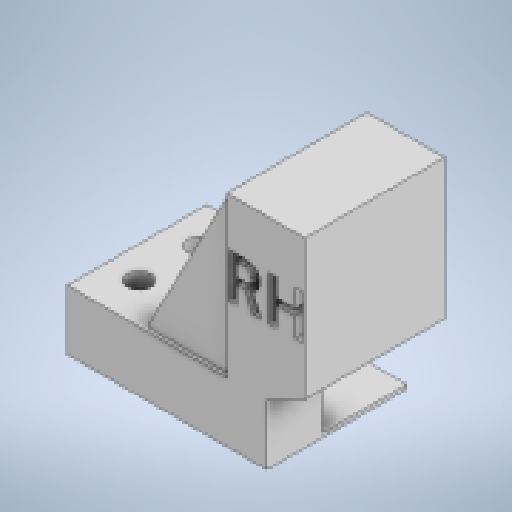
# Autodesk Inventor part: gripper
Saved by Autodesk Inventor 2024 (Build 280153000, 153)
## iProperties
Created: 2023-09-08
Part Number: gripper
Material: Generic
Document SubType Name: Modeling
Designer: 박동준
Density: 1 g/cm^3
Appearance: Default
Author: 박동준
Autodesk Inventor part; units mm, degrees
ref_plane "YZ Plane" through (0, 0, 0) normal (1, 0, 0) x (0, 1, 0)
ref_plane "XZ Plane" through (0, 0, 0) normal (0, 1, 0) x (-1, 0, 0)
sketch "Sketch1" plane through (0, 0, 0) normal (0, 0, 1) x (1, 0, 0)
  line L0 (-10, 40) -> (-10, 0)
  line L1 (-10, 0) -> (0, 0)
  line L2 (0, 0) -> (9.5, 5)
  line L3 (9.5, 5) -> (9.5, 40)
  line L4 (9.5, 40) -> (-10, 40)
  dimension "d0" = 40
  dimension "d2" = 10
  dimension "d55" = 9.5
  dimension "d57" = 35
  constraints: 10 end point, 2 perpendicular, 1 parallel, 1 vertical
  measures "d0" distance of L0.start L0.end
  measures "d2" distance of L0.end L1.end
  measures "d55" distance from line of L3 L1.end
  measures "d57" distance of L2.end L3.end
extrude "Extrusion1" add sketch "Sketch1" along normal mid plane 35
ref_plane "Work Plane1" through (0, 0, 15) normal (0, 0, 1) x (1, 0, 0)
sketch "Sketch2" plane through (0, 0, 15) normal (0, 0, 1) x (1, 0, 0)
  line L0 (-10, 40) -> (-10, 0) projected
  line L1 (-10, 0) -> (0, 0) projected
  line L2 (-10, 0) -> (-31, 0)
  line L3 (-10, 0) -> (11, 0) construction
  line L4 (0, 0) -> (9.5, 5) projected
  line L5 (9.5, 5) -> (9.5, 40) projected
  line L6 (9.5, 40) -> (-10, 40) projected
  line L7 (-31, 0) -> (-10, 40)
  line L8 (-10, 0) -> (-10, 40)
  dimension "d9" = 21
  dimension "d10" = 180
  dimension "d88" = 40
  constraints: 8 end point, 2 collinear, 2 horizontal, 1 point on line
  measures "d9" distance of L0.end L2.end
  measures "d10" angle of L2 L3
  measures "d88" distance from line of L1 L7.end
extrude "Extrusion2" add sketch "Sketch2" along normal mid plane 3 contours L0 L2 L7
mirror "Mirror1" about plane through (0, 0, 0) normal (0, 0, 1) of "Extrusion2"
sketch "Sketch3" plane through (-10, 0, 17.5) normal (0, -1, 0) x (1, 0, 0)
  line L0 (-40, 2) -> (-15.2727, 11)
  line L1 (-15.2727, 11) -> (10, 11)
  line L2 (10, 11) -> (10, -46)
  line L3 (-40, 2) -> (-40, -37)
  line L4 (-40, -37) -> (-15.2727, -46)
  line L5 (-15.2727, -46) -> (10, -46)
  line L6 (10, -35) -> (10, 0) projected
  line L7 (10, -35) -> (10, 0) projected
  line L8 (0, 0) -> (0, -1) projected
  line L9 (10, -35) -> (0, -35) projected
  line L10 (0, 0) -> (10, 0) projected
  line L11 (-21, -1) -> (0, -1) projected
  line L12 (-21, -4) -> (-21, -1) projected
  line L13 (0, -4) -> (-21, -4) projected
  line L14 (0, -4) -> (0, -31) projected
  line L15 (0, -31) -> (-21, -31) projected
  line L16 (-21, -31) -> (-21, -34) projected
  line L17 (-21, -34) -> (0, -34) projected
  line L18 (0, -34) -> (0, -35) projected
  point P0 (10, -17.5)
  point P1 (-2.6364, 11)
  point P2 (10, -17.5)
  point P3 (10, -17.5)
  point P4 (10, -17.5)
  point P5 (-2.6364, -46)
  point P6 (-40, -17.5)
  point P7 (10, -17.5)
  point P8 (10, -35)
  point P9 (10, 0)
  dimension "d17" = 57
  dimension "d18" = 39
  dimension "d19" = 9
  dimension "d20" = 9
  dimension "d21" = 50
  dimension "d76" = 110
  constraints: 12 end point, 7 midpoint, 3 coincident, 1 horizontal alignment, 1 perpendicular, 1 vertical alignment
  measures "d17" distance of L1.end L2.end
  measures "d18" distance of L0.start L3.end
  measures "d19" distance from line of L5 L3.end
  measures "d20" vertical distance of point (-2.636, 11) L0.start
  measures "d21" distance between parallel lines of L2 L3
  measures "d76" angle of L3 L4
extrude "Extrusion3" add sketch "Sketch3" along normal blind 15
sketch "Sketch4" plane through (-10, 0, 17.5) normal (0, 1, 0) x (1, 0, 0)
  line L0 (10, 17.5) -> (-48, 17.5) construction
  line L1 (-32, 10) -> (-12, 10) construction
  line L2 (-32, 25) -> (-32, 10) construction
  line L3 (10, 35) -> (0, 35) projected
  line L4 (10, 46) -> (10, 35) projected
  line L5 (-15.2727, 46) -> (10, 46) projected
  line L6 (-40, 37) -> (-15.2727, 46) projected
  line L7 (-40, -2) -> (-40, 37) projected
  line L8 (-15.2727, -11) -> (-40, -2) projected
  line L9 (10, -11) -> (-15.2727, -11) projected
  line L10 (10, 0) -> (10, -11) projected
  line L11 (0, 0) -> (10, 0) projected
  line L12 (0, 0) -> (0, 1) projected
  line L13 (-21, 1) -> (0, 1) projected
  line L14 (-21, 4) -> (-21, 1) projected
  line L15 (0, 4) -> (-21, 4) projected
  line L16 (0, 4) -> (0, 31) projected
  line L17 (0, 31) -> (-21, 31) projected
  line L18 (-21, 31) -> (-21, 34) projected
  line L19 (-21, 34) -> (0, 34) projected
  line L20 (0, 34) -> (0, 35) projected
  point P0 (-32, 17.5)
  point P1 (-19, 17.5)
  dimension "d26" = 20
  dimension "d27" = 15
  dimension "d58" = 13
  dimension "d59" = 8
  constraints: 6 end point, 2 horizontal, 2 midpoint, 2 perpendicular, 1 horizontal alignment
  measures "d26" distance of L1.end L1.start
  measures "d27" distance of L2.start L1.start
  measures "d58" distance from line of L2 point (-19, 17.5)
  measures "d59" distance from line of point (-32, 17.5) L7
hole "Hole1" at (-42, 0, 7.5) at (-22, 0, 7.5) at (-42, 0, -7.5) direction (0, -1, 0) diameter 3.1 end through all
sketch "Sketch5" plane through (0, 0, -17.5) normal (1, 0, 0) x (0, 0, -1)
  line L0 (11, 0) -> (0, 0) projected
  line L1 (-35, 0) -> (-46, 0) projected
  line L2 (-46, 0) -> (-46, -15) projected
  line L3 (11, -15) -> (-46, -15) projected
  line L4 (11, 0) -> (11, -15) projected
  line L5 (-46, 0) -> (-46, -15) projected
  line L6 (-21, -4) -> (9, -4)
  line L7 (9, -4) -> (9, -14)
  line L8 (9, -14) -> (-21, -14)
  line L9 (-21, -14) -> (-21, -4)
  line L10 (0, 0) -> (-35, 0) projected
  point P0 (-17.5, 0)
  point P1 (-17.5, 0)
  point P2 (-46, -7.5)
  point P3 (-46, -7.5)
  point P4 (11, -12.5)
  point P5 (11, -2.5)
  dimension "d46" = 30
  dimension "d47" = 10
  dimension "d48" = 2
  dimension "d49" = 4
  constraints: 8 end point, 2 midpoint, 2 parallel
  measures "d46" distance of L7.end L8.end
  measures "d47" distance of L6.end L7.end
  measures "d48" distance between parallel lines of L4 L7
  measures "d49" distance between parallel lines of L6 L0
extrude "Extrusion4" cut sketch "Sketch5" against normal blind 30 contours L6 L7 L8 L9
sketch "Sketch6" plane through (-10, 0, 17.5) normal (0, 1, 0) x (1, 0, 0)
  circle A0 centre (-32, 25) radius 1.55 projected
  circle A1 centre (-12, 10) radius 1.55 projected
  circle A2 centre (-32, 10) radius 1.55 projected
  line L0 (10, 35) -> (0, 35) projected
  line L1 (10, 46) -> (10, 35) projected
  line L2 (-15.2727, 46) -> (10, 46) projected
  line L3 (-40, 37) -> (-15.2727, 46) projected
  line L4 (-40, -2) -> (-40, 37) projected
  line L5 (-15.2727, -11) -> (-40, -2) projected
  line L6 (10, -11) -> (-15.2727, -11) projected
  line L7 (10, 0) -> (10, -11) projected
  line L8 (0, 0) -> (10, 0) projected
  line L9 (0, 0) -> (0, 1) projected
  circle A3 centre (-12, 25) radius 2.9
  line L10 (-21, 1) -> (0, 1) projected
  line L11 (-21, 4) -> (-21, 1) projected
  line L12 (0, 4) -> (-21, 4) projected
  line L13 (0, 4) -> (0, 31) projected
  line L14 (0, 31) -> (-21, 31) projected
  line L15 (-21, 31) -> (-21, 34) projected
  line L16 (-21, 34) -> (0, 34) projected
  line L17 (0, 34) -> (0, 35) projected
  point P0 (10, 17.5)
  dimension "d41" = 5.8
  dimension "d42" = 20
  dimension "d43" = 15
  constraints: 1 centre point
  measures "d41" diameter of A3
  measures "d42" distance of A3.centre A0.centre
  measures "d43" distance of A3.centre A1.centre
extrude "Extrusion5" cut sketch "Sketch6" against normal blind 3 contours A3
sketch "Sketch7" plane through (-10, -15, 17.5) normal (0, -1, 0) x (1, 0, 0)
  circle A0 centre (-12, -25) radius 1.55
  circle A1 centre (-32, -25) radius 1.55 projected
  circle A2 centre (-12, -10) radius 1.55 projected
  circle A3 centre (-32, -10) radius 1.55 projected
  line L0 (10, -46) -> (10, 11) projected
  line L1 (10, 11) -> (-15.2727, 11) projected
  line L2 (-15.2727, 11) -> (-40, 2) projected
  line L3 (-40, 2) -> (-40, -37) projected
  line L4 (-40, -37) -> (-15.2727, -46) projected
  line L5 (-15.2727, -46) -> (10, -46) projected
  point P0 (10, -17.5)
  dimension "d50" = 15
  dimension "d51" = 20
  dimension "d52" = 3.1
  constraints: 1 centre point
  measures "d50" distance of A0.centre A2.centre
  measures "d51" distance of A1.centre A0.centre
  measures "d52" diameter of A0
extrude "Extrusion6" cut sketch "Sketch7" against normal up to surface (1 mm away) contours A0
sketch "Sketch8" plane through (0, 0, 17.5) normal (0, 0, 1) x (1, 0, 0)
  line L0 (-10, 0) -> (0, 0) projected
  line L1 (0, 0) -> (9.5, 5) projected
  line L2 (9.5, 5) -> (9.5, 40) projected
  line L3 (9.5, 40) -> (-10, 40) projected
  line L4 (-10, 40) -> (-10, 0) projected
  line L5 (-10.7901, 28) -> (5, 28) construction
  line L6 (5, 28) -> (5, 11.9362) construction
  line L7 (5, 11.9362) -> (-10.7901, 11.9362) construction
  line L8 (-10.7901, 11.9362) -> (-10.7901, 28) construction
  line L9 (-5.3559, 21.4049) -> (-7.6037, 21.4049)
  line L10 (-7.6037, 21.4049) -> (-7.6037, 17)
  line L11 (-7.6037, 17) -> (-9.555, 17)
  line L12 (-9.555, 17) -> (-9.555, 28)
  line L13 (-9.555, 28) -> (-5.3889, 28)
  spline S0 degree 2 poles (-5.3889, 28) (-4.5326, 28) (-3.207, 27.5389) (-2.3095, 26.7485) (-1.832, 25.637) (-1.832, 24.9783) knots 0 0 0 1 2 3 4 4 4
  line L14 (-1.832, 24.9783) -> (-1.832, 24.4102)
  spline S1 degree 2 poles (-1.832, 24.4102) (-1.832, 23.5457) (-2.6883, 22.1542) (-3.5445, 21.7754) knots 0 0 0 1 2 2 2
  spline S2 degree 2 poles (-3.5445, 21.7754) (-2.9929, 20.5651) (-1.939, 18.2021) (-1.3956, 17) knots 0 0 0 1 2 2 2
  line L15 (-1.3956, 17) -> (-3.5116, 17)
  line L16 (-3.5116, 17) -> (-5.3559, 21.4049)
  line L17 (-7.6037, 26.3698) -> (-7.6037, 23.0434)
  line L18 (-7.6037, 23.0434) -> (-5.8005, 23.0434)
  spline S3 degree 2 poles (-5.8005, 23.0434) (-4.6725, 23.0434) (-3.7751, 23.8338) (-3.7751, 24.4596) knots 0 0 0 1 2 2 2
  line L19 (-3.7751, 24.4596) -> (-3.7751, 24.9207)
  spline S4 degree 2 poles (-3.7751, 24.9207) (-3.7751, 25.5546) (-4.6231, 26.3698) (-5.6359, 26.3698) knots 0 0 0 1 2 2 2
  line L20 (-5.6359, 26.3698) -> (-7.6037, 26.3698)
  line L21 (7.0273, 21.9237) -> (2.4659, 21.9237)
  line L22 (2.4659, 21.9237) -> (2.4659, 17)
  line L23 (2.4659, 17) -> (0.5146, 17)
  line L24 (0.5146, 17) -> (0.5146, 28)
  line L25 (0.5146, 28) -> (2.4659, 28)
  line L26 (2.4659, 28) -> (2.4659, 23.5457)
  line L27 (2.4659, 23.5457) -> (7.0273, 23.5457)
  line L28 (7.0273, 23.5457) -> (7.0273, 28)
  line L29 (7.0273, 28) -> (8.9869, 28)
  line L30 (8.9869, 28) -> (8.9869, 17)
  line L31 (8.9869, 17) -> (7.0273, 17)
  line L32 (7.0273, 17) -> (7.0273, 21.9237)
  point P0 (-7, 15)
  dimension "d68" = 12
  dimension "d69" = 15
  constraints: 2 other
  measures "d68" distance between parallel lines of L5 L3
  measures "d69" distance between parallel lines of L6 L4
extrude "Extrusion7" cut sketch "Sketch8" against normal blind 5 contours L9 L10 L11 L12 L13 S0 L14 S1 S2 L15 L16 | L21 L22 L23 L24 L25 L26 L27 L28 L29 L30 L31 L32
sketch "Sketch9" plane through (0, 0, -17.5) normal (0, 0, -1) x (-1, 0, 0)
  line L0 (-0.5146, 17) -> (-0.5146, 28) projected
  line L1 (0, 0) -> (10, 0) projected
  line L2 (10, 0) -> (10, 40) projected
  line L3 (10, 40) -> (-9.5, 40) projected
  line L4 (-9.5, 40) -> (-9.5, 5) projected
  line L5 (-9.5, 5) -> (0, 0) projected
  line L6 (-7.3088, 28) -> (-3.8059, 28) construction
  line L7 (-3.8059, 28) -> (-3.8059, 25.5662) construction
  line L8 (-3.8059, 25.5662) -> (-7.3088, 25.5662) construction
  line L9 (-7.3088, 25.5662) -> (-7.3088, 28) construction
  line L10 (5.5, 50.4054) -> (5.5, 41.2692)
  line L11 (6.1232, 21.3023) -> (1.0421, 21.3023)
  line L12 (1.0421, 21.3023) -> (1.0421, 16.2212)
  line L13 (1.0421, 16.2212) -> (-0.6353, 16.2212)
  line L14 (-0.6353, 16.2212) -> (-0.6353, 21.3023)
  line L15 (-0.6353, 21.3023) -> (-5.7164, 21.3023)
  line L16 (-5.7164, 21.3023) -> (-5.7164, 22.919)
  line L17 (-5.7164, 22.919) -> (-0.6353, 22.919)
  line L18 (-0.6353, 22.919) -> (-0.6353, 28)
  line L19 (-0.6353, 28) -> (1.0421, 28)
  line L20 (1.0421, 28) -> (1.0421, 22.919)
  line L21 (1.0421, 22.919) -> (6.1232, 22.919)
  line L22 (6.1232, 22.919) -> (6.1232, 21.3023)
  dimension "d72" = 12
  dimension "d73" = 15
  constraints: 2 end point, 1 vertical, 2 other
  measures "d72" distance between parallel lines of L3 L6
  measures "d73" distance between parallel lines of L10 L4
extrude "Extrusion8" cut sketch "Sketch9" against normal blind 5 contours L11 L12 L13 L14 L15 L16 L17 L18 L19 L20 L21 L22
sketch "Sketch10" plane through (-10, 0, 17.5) normal (0, 1, 0) x (1, 0, 0)
  line L0 (-39.35, 19.5) -> (-4.65, 19.5) projected
  circle A0 centre (-32, 25) radius 1.55 projected
  circle A1 centre (-32, 10) radius 1.55 projected
  circle A2 centre (-12, 10) radius 1.55 projected
  circle A3 centre (-32, 25) radius 2.9
  circle A4 centre (-32, 10) radius 2.9
  circle A5 centre (-12, 10) radius 2.9
  point P0 (10, 17.5)
  dimension "d77" = 5.8
  dimension "d78" = 5.8
  dimension "d79" = 5.8
  constraints: 3 centre point, 3 coincident
  measures "d77" diameter of A3
  measures "d78" diameter of A4
  measures "d79" diameter of A5
extrude "Extrusion9" cut sketch "Sketch10" against normal blind 10 contours A0 | A1 | A3 | A4 | A5
sketch "Sketch12" plane through (-10, 0, 17.5) normal (0, 1, 0) x (1, 0, 0)
  circle A0 centre (-12, 25) radius 2.9 projected
  circle A1 centre (-12, 25) radius 1.55
  point P0 (10, 17.5)
  dimension "d85" = 3.1
  constraints: 2 coincident, 1 centre point
  measures "d85" diameter of A1
extrude "Extrusion11" cut sketch "Sketch12" against normal blind 4 contours A1
sketch "Sketch13" plane through (-10, 0, 17.5) normal (0, 1, 0) x (1, 0, 0)
  circle A0 centre (-12, 10) radius 2.9 projected
  circle A1 centre (-32, 25) radius 2.9 projected
  circle A2 centre (-32, 10) radius 2.9 projected
  circle A3 centre (-12, 25) radius 2.9 projected
  line L0 (10, 35) -> (0, 35) projected
  line L1 (10, 46) -> (10, 35) projected
  line L2 (-15.2727, 46) -> (10, 46) projected
  line L3 (-40, 37) -> (-15.2727, 46) projected
  line L4 (-40, -2) -> (-40, 37) projected
  line L5 (-15.2727, -11) -> (-40, -2) projected
  line L6 (10, -11) -> (-15.2727, -11) projected
  line L7 (10, 0) -> (10, -11) projected
  line L8 (0, 0) -> (10, 0) projected
  line L9 (0, 0) -> (0, 1) projected
  line L10 (-21, 1) -> (0, 1) projected
  line L11 (-21, 4) -> (-21, 1) projected
  line L12 (0, 4) -> (-21, 4) projected
  line L13 (0, 4) -> (0, 31) projected
  line L14 (0, 31) -> (-21, 31) projected
  line L15 (-21, 31) -> (-21, 34) projected
  line L16 (-21, 34) -> (0, 34) projected
  line L17 (0, 34) -> (0, 35) projected
  line L18 (10, -11) -> (-40, -11)
  line L19 (-40, -11) -> (-40, 0)
  line L20 (-40, 0) -> (10, 0)
  line L21 (10, 0) -> (10, -11)
  line L22 (10, 46) -> (-40, 46)
  line L23 (-40, 46) -> (-40, 35)
  line L24 (-40, 35) -> (10, 35)
  line L25 (10, 35) -> (10, 46)
  point P0 (10, 17.5)
  point P1 (10, 40.5)
  point P2 (-40, 35)
  dimension "d89" = 11
  dimension "d92" = 11
  dimension "d93" = 50
  constraints: 16 end point, 4 parallel, 2 horizontal, 2 perpendicular, 1 midpoint, 1 point on line
  measures "d89" distance between parallel lines of L18 L20
  measures "d92" distance between parallel lines of L2 L24
  measures "d93" distance from line of point (10, 40.5) L23
extrude "Extrusion12" cut sketch "Sketch13" against normal blind 30 contours L0 L24 L4 L3 L2 L1 | L20 L8 L7 L6 L5 L4
body "Solid1"
